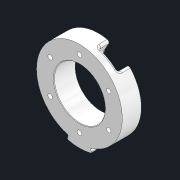
# Autodesk Inventor part: base9_2
Saved by Autodesk Inventor 2022 (Build 260153000, 153)
## iProperties
Created: 2021-07-25
Part Number: base9_2
Material: ABS プラスチック
Document SubType Name: Modeling
Designer: yuto6
Density: 1.06 g/cm^3
Appearance: 滑らか - 白
Mass: 25.5038 g
Surface Area: 104.746 cm^2
Volume: 24.0602 cm^3
購入先: 印刷
在庫数: 0.0
Author: yuto6
Autodesk Inventor part; units mm, degrees
ref_plane "YZ Plane" through (0, 0, 0) normal (1, 0, 0) x (0, 1, 0)
ref_plane "XZ Plane" through (0, 0, 0) normal (0, 1, 0) x (-1, 0, 0)
ref_plane "XY Plane" through (0, 0, 0) normal (0, 0, 1) x (1, 0, 0)
sketch "スケッチ2" plane through (0, 0, 0) normal (1, 0, 0) x (0, 1, 0)
  line L0 (24.1, 0) -> (24.1, -20)
  line L1 (40.5, 0) -> (40.5, -18)
  line L2 (40.5, 0) -> (24.1, 0)
  line L3 (24.1, 0) -> (59, 0)
  line L4 (24.1, -20) -> (28, -20)
  line L5 (0, -24) -> (0, 4) projected
  line L6 (28, -20) -> (28, -18)
  line L7 (28, -18) -> (40.5, -18)
  point P0 (0, 0)
  dimension "d40" = 24.1
  dimension "d41" = 18
  dimension "d42" = 40.5
  dimension "d43" = 28
  dimension "d44" = 2
  constraints: 14 end point, 3 horizontal, 3 perpendicular, 1 horizontal alignment, 1 vertical
  measures "d40" distance from line of point (0, 0) L0
  measures "d41" distance of L1.end L1.start
  measures "d42" distance from line of point (0, 0) L1
  measures "d43" distance between parallel lines of L5 L6
  measures "d44" distance of L4.end L6.end
revolve "回転1" add sketch "スケッチ2" angle 360 about axis through (0, 0, -10) along (0, 0, 1)
sketch "スケッチ4" plane through (0, 0, 0) normal (0, 0, 1) x (1, 0, 0)
  point P0 (0, 0)
  point P1 (0, 32)
  point P2 (-27.7128, 16)
  point P3 (-27.7128, -16)
  point P4 (0, -32)
  point P5 (27.7128, -16)
  point P6 (27.7128, 16)
  dimension "d11" = 32
  dimension "d14" = 360
  constraints: 7 other
  measures "d11" distance of point (0, 0) point (0, 32)
hole "穴1" at (0, 32, 0) at (-27.7128, 16, 0) at (-27.7128, -16, 0) at (0, -32, 0) at (27.7128, -16, 0) at (27.7128, 16, 0) direction (0, 0, -1) diameter 4.3 end through all clearance for "Socket Head Cap Screw" size "M4" standard "Ansi Metric M Profile"
chamfer "面取り3" distance 0.5 angle 45 1 edges at (0, -28, -20)
chamfer "面取り4" distance 0.5 angle 45 1 edges at (0, -24.1, 0)
sketch "スケッチ7" plane through (0, 0, 0) normal (0, 0, 1) x (1, 0, 0)
  circle A0 centre (0, 0) radius 40.5 projected
  circle A1 centre (0, 0) radius 44.5
  line L0 (0, 0) -> (11.5174, -42.9837)
  line L1 (0, 0) -> (-11.5174, -42.9837)
  line L2 (0, 62.3) -> (0, -62.3) projected
  point P0 (10.4822, -39.12)
  point P1 (-10.4822, -39.12)
  dimension "d51" = 4
  dimension "d52" = 15
  dimension "d53" = 15
  constraints: 4 end point, 2 point on circle, 1 centre point
  measures "d51" radial gap between concentric circles of A0 A1
  measures "d52" angle of L2 L0
  measures "d53" angle of L2 L1
extrude "押し出し3" add sketch "スケッチ7" against normal blind 5 contours L0 A1 L2 A0 | A0 L2 A1 L1 picked at (6.2128, -42.6798) picked at (-1.2928, -43.1102)
fillet "フィレット1" radius 1 4 edges at (10.4822, -39.12, -2.5) (11.5174, -42.9837, -2.5) (-10.4822, -39.12, -2.5) (-11.5174, -42.9837, -2.5)
sketch "スケッチ8" plane through (0, 0, -20) normal (0, 0, -1) x (-1, 0, 0)
  line L0 (0, 0) -> (-24.0103, 41.587)
  circle A0 centre (0, 0) radius 40.5 projected
  circle A1 centre (0, 0) radius 24.1 projected
  line L1 (0, -57.9174) -> (0, 64.0044) projected
  line L2 (-8.6603, -5) -> (-32.6705, 36.587)
  line L3 (8.6603, 5) -> (-15.35, 46.587)
  point P0 (-2.3034, 23.9897)
  point P1 (-10.9628, 38.988)
  point P2 (-28.2833, 28.988)
  point P3 (-19.6239, 13.9897)
  dimension "d57" = 210
  dimension "d58" = 10
  dimension "d59" = 10
  constraints: 6 end point, 2 parallel
  measures "d58" distance between parallel lines of L0 L2
  measures "d59" distance between parallel lines of L0 L3
extrude "押し出し4" cut sketch "スケッチ8" against normal blind 12 contours A1 L2 A0 L0 | L0 A0 L3 A1
fillet "フィレット2" radius 2 2 edges at (6.6331, 31.4889, -8) (23.9536, 21.4889, -8)
fillet "フィレット3" radius 2 6 edges at (28.2833, 28.988, -14) (11.4568, 38.8458, -8.6783) (10.9628, 38.988, -14) (2.869, 23.9286, -8.6545) (19.6239, 13.9897, -15) (2.3034, 23.9897, -15)
equation "\"d59\" = d58"
